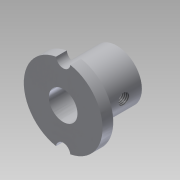
# Autodesk Inventor part: Raccord-Mat-Potence
Saved by Autodesk Inventor 2016 (Build 200138000, 138)
## iProperties
Created: 2016-01-27
Part Number: Raccord-Mat-Potence
Material: Aluminium 6061
Document SubType Name: Modeling
Designer: sd
Density: 2.71 g/cm^3
Appearance: Aluminium - Plat
Author: sd
Autodesk Inventor part; units mm, degrees
ref_plane "XZ Plane" through (0, 0, 0) normal (0, 1, 0) x (-1, 0, 0)
ref_plane "XY Plane" through (0, 0, 0) normal (0, 0, 1) x (1, 0, 0)
sketch "Esquisse1" plane through (0, 0, 0) normal (0, 1, 0) x (-1, 0, 0)
  circle A0 centre (0, 0) radius 11
  dimension "d0" = 22
  constraints: 1 centre point, 1 coincident
  measures "d0" diameter of A0
extrude "Extrusion1" add sketch "Esquisse1" along normal blind 15
sketch "Esquisse2" plane through (0, 15, 0) normal (0, 1, 0) x (1, 0, 0)
  circle A0 centre (0, 0) radius 11 projected
  circle A1 centre (0, 0) radius 7
  dimension "d3" = 14
  constraints: 1 centre point, 1 coincident
  measures "d3" diameter of A1
extrude "Extrusion2" cut sketch "Esquisse2" against normal blind 12
sketch "Esquisse3" plane through (0, 15, 0) normal (0, 1, 0) x (1, 0, 0)
  circle A0 centre (0, 0) radius 7 projected
  circle A1 centre (0, 0) radius 4
  dimension "d6" = 8
  constraints: 1 centre point, 1 coincident
  measures "d6" diameter of A1
extrude "Extrusion3" cut sketch "Esquisse3" against normal through all contours A1
sketch "Esquisse4" plane through (0, 0, 0) normal (0, -1, 0) x (1, 0, 0)
  circle A0 centre (0, 0) radius 11 projected
  circle A1 centre (0, 11) radius 2
  circle A2 centre (0, -11) radius 2
  dimension "d9" = 4
  dimension "d10" = 4
  constraints: 2 centre point, 2 point on circle
  measures "d9" diameter of A1
  measures "d10" diameter of A2
extrude "Extrusion4" cut sketch "Esquisse4" against normal through all contours A1 A0 | A0 A1 | A2 A0 | A0 A2
ref_plane "Plan de construction1" through (7, 15, 0) normal (1, 0, 0) x (0, 1, 0)
sketch "Esquisse5" plane through (7, 15, 0) normal (1, 0, 0) x (0, 1, 0)
  circle A0 centre (-5, 0) radius 1.5
  line L0 (0, -7) -> (0, 7) projected
  point P0 (-15, 0)
  dimension "d13" = 3
  dimension "d16" = 5
  constraints: 1 centre point
  measures "d13" diameter of A0
  measures "d16" distance from line of L0 A0.centre
extrude "Extrusion5" cut sketch "Esquisse5" against normal blind 5
thread "Filetage1" size "M3x0.5" class "6H" standard "ANSI Metric M Profile" full length
equation "\"d10\" = d9"
